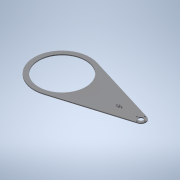
# Autodesk Inventor part: ForeArm_inside_frame
Saved by Autodesk Inventor 2020.4 (Build 244396000, 396)
## iProperties
Created: 2016-05-04
Part Number: ForeArm_inside_frame
Material: GFRP
Document SubType Name: Modeling
Designer: hiroaki
Density: 1.75 g/cm^3
Appearance: 滑らか - 淡い灰色
Mass: 3.24569 g
Surface Area: 24.0552 cm^2
Volume: 1.85468 cm^3
Description: GFRP T2
d0: 147.500 mm
d1: 3.100 mm
d2: 21.000 mm
d3: 10.000 mm
d4: 5.000 mm
d5: 12.000 mm
d6: 100.000 mm
d7: 5.000 mm
d8: 0.050 mm
d9: 2.100 mm
d10: 2.700 mm
d11: 8.500 mm
d12: 10.100 mm
d13: 4.000 ul
d15: 360.00 deg
d17: 2.000 mm
d18: 0.00 deg
Author: hiroaki
Autodesk Inventor part; units mm, degrees
ref_plane "YZ Plane" through (0, 0, 0) normal (1, 0, 0) x (0, 1, 0)
ref_plane "XZ Plane" through (0, 0, 0) normal (0, 1, 0) x (-1, 0, 0)
ref_plane "XY Plane" through (0, 0, 0) normal (0, 0, 1) x (1, 0, 0)
sketch "スケッチ1" plane through (0, 0, 0) normal (0, 0, 1) x (1, 0, 0)
  circle A0 centre (0, 0) radius 10.5 construction
  line L0 (0, 10.5) -> (-147.5, 10.5) construction
  line L1 (-147.5, 10.5) -> (-147.5, -10.5) construction
  line L2 (-147.5, -10.5) -> (0, -10.5) construction
  circle A1 centre (-142.5, 0) radius 1.55 construction
  line L3 (-132.5, 2.5) -> (-52.5, 2.5) construction
  line L4 (-52.5, 2.5) -> (-52.5, -2.5) construction
  line L5 (-52.5, -2.5) -> (-132.5, -2.5) construction
  line L6 (-132.5, -2.5) -> (-132.5, 2.5) construction
  line L7 (-92.5, 2.5) -> (-92.5, -2.5) construction
  circle A2 centre (-42.5, 0) radius 1.55 construction
  line L8 (-12, 21.3027) -> (-12, -27.3903) construction
  line L9 (-52.45, 2.55) -> (-132.55, 2.55) construction
  line L10 (-132.55, 2.55) -> (-132.55, -2.55) construction
  line L11 (-132.55, -2.55) -> (-52.45, -2.55) construction
  line L12 (-52.45, -2.55) -> (-52.45, 2.55) construction
  circle A3 centre (-131.5, 2.55) radius 1.05 construction
  line L13 (-132.5, 0) -> (-92.5, 0) construction
  line L14 (-132.55, 2.55) -> (-132.55, -2.55) construction
  arc A4 (-130.45, 2.55) -> (-132.55, 2.55) centre (-131.5, 2.55) ccw construction
  line L15 (-130.45, 2.55) -> (-54.55, 2.55) construction
  arc A5 (-52.45, 2.55) -> (-54.55, 2.55) centre (-53.5, 2.55) ccw construction
  line L16 (-52.45, 2.55) -> (-52.45, -2.55) construction
  arc A6 (-132.55, -2.55) -> (-130.45, -2.55) centre (-131.5, -2.55) ccw construction
  line L17 (-130.45, -2.55) -> (-54.55, -2.55) construction
  arc A7 (-54.55, -2.55) -> (-52.45, -2.55) centre (-53.5, -2.55) ccw construction
  circle A8 centre (0, 8.5) radius 1.35
  circle A9 centre (0, 0) radius 5.05
  circle A10 centre (-8.5, 0) radius 1.35
  circle A11 centre (0, -8.5) radius 1.35
  circle A12 centre (8.5, 0) radius 1.35
  line L18 (-147.5, 4.7329) -> (-147.5, -4.7329) construction
  line L19 (-147.5, 4.7329) -> (-42.5, 10.5) construction
  line L20 (-42.5, 10.5) -> (0, 10.5) construction
  line L21 (-147.5, -4.7329) -> (-42.5, -10.5) construction
  line L22 (-42.5, -10.5) -> (0, -10.5) construction
  arc A13 (0, -10.5) -> (0, 10.5) centre (0, 0) ccw construction
  circle A14 centre (-142.5, 0) radius 5 construction
  circle A15 centre (-41.5, 0) radius 1.55
  circle A16 centre (-51.5, 0) radius 1.55
  line L23 (-37.5, -2.5) -> (-55.5, -2.5) construction
  line L24 (-55.5, -2.5) -> (-55.5, 2.5) construction
  line L25 (-55.5, 2.5) -> (-37.5, 2.5) construction
  line L26 (-37.5, 2.5) -> (-37.5, -2.5) construction
  line L27 (-47.5, -2.5) -> (-45.5, -2.5) construction
  line L28 (-45.5, -2.5) -> (-45.5, 2.5) construction
  line L29 (-45.5, 2.5) -> (-47.5, 2.5) construction
  line L30 (-47.5, 2.5) -> (-47.5, -2.5) construction
  line L31 (-47.45, -2.55) -> (-45.55, -2.55)
  line L32 (-45.55, -2.55) -> (-45.55, 2.55)
  line L33 (-45.55, 2.55) -> (-47.45, 2.55)
  line L34 (-47.45, 2.55) -> (-47.45, -2.55)
  circle A17 centre (-48.5, -2.55) radius 1.05
  circle A18 centre (-48.5, 2.55) radius 1.05
  circle A19 centre (-44.5, -2.55) radius 1.05
  circle A20 centre (-44.5, 2.55) radius 1.05
  line L35 (-55.5, 2.5) -> (-55.5, -2.5)
  line L36 (-55.5, -2.5) -> (-21.9113, -10.5)
  line L37 (-55.5, 2.5) -> (-21.9113, 10.5)
  arc A21 (0, -10.5) -> (0, 10.5) centre (0, 0) ccw
  line L38 (-21.9113, 10.5) -> (0, 10.5)
  line L39 (0, -10.5) -> (-21.9113, -10.5)
  circle A22 centre (-44.5, 2.55) radius 2.5 construction
  circle A23 centre (0, 0) radius 16 construction
  circle A24 centre (0, 0) radius 21 construction
  line L40 (-21, 19.3585) -> (-21, -28.09) construction
  circle A25 centre (-169.122, 0) radius 50.4075
  circle A26 centre (-169.122, 0) radius 60
  line L41 (-151.5607, 57.3725) -> (3.0732, 10.0402)
  line L42 (-151.5607, -57.3725) -> (3.0732, -10.0402)
  point P0 (-147.5, 0)
  point P1 (-37.5, 0)
  point P2 (3.0732, -10.0402)
  dimension "d9" = 2.1
  dimension "d29" = 2.1
  dimension "d36" = 120
  dimension "d0" = 147.5
  dimension "d1" = 3.1
  dimension "d2" = 21
  dimension "d3" = 10
  dimension "d4" = 5
  dimension "d5" = 12
  dimension "d6" = 100
  dimension "d7" = 5
  dimension "d8" = 0.05
  dimension "d10" = 2.7
  dimension "d11" = 8.5
  dimension "d12" = 10.1
  dimension "d15" = 360
  dimension "d20" = 3.1
  dimension "d21" = 5
  dimension "d22" = 4
  dimension "d23" = 5
  dimension "d24" = -10
  dimension "d26" = 10
  dimension "d27" = 4
  dimension "d28" = 10
  dimension "d30" = 0.05
  dimension "d32" = 5
  dimension "d33" = 32
  dimension "d34" = 5
  dimension "d35" = 100.815
  dimension "d37" = 169.122
  constraints: 86 end point, 20 centre point, 15 point on circle, 12 tangent, 11 horizontal alignment, 10 coincident, 10 parallel, 9 horizontal, 8 perpendicular, 7 midpoint, 7 symmetric about line, 6 point on line, 5 collinear, 5 vertical, 4 equal radius, 3 vertical alignment, 2 concentric, 34 other
  measures "d0" distance from line of L1 point (0, 0)
  measures "d1" diameter of A1
  measures "d2" distance of L0.end L1.end
  measures "d3" distance from line of L6 A1.centre
  measures "d4" distance from line of L1 A1.centre
  measures "d5" distance from line of point (0, 0) L8
  measures "d6" distance of A2.centre A1.centre
  measures "d7" distance of L3.end L4.end
  measures "d8" distance between parallel lines of L9 L3
  measures "d10" diameter of A8
  measures "d11" distance of point (0, 0) A8.centre
  measures "d12" diameter of A9
  measures "d20" diameter of A15
  measures "d21" distance from line of L26 A2.centre
  measures "d22" distance from line of L26 A15.centre
  measures "d23" distance of L25.end L23.start
  measures "d24" distance of A16.centre A15.centre
  measures "d26" distance between parallel lines of L30 L26
  measures "d27" distance from line of A16.centre L24
  measures "d28" distance between parallel lines of L28 L24
  measures "d30" distance between parallel lines of L34 L30
  measures "d32" diameter of A22
  measures "d33" diameter of A23
  measures "d34" radial gap between concentric circles of A24 A23
  measures "d35" diameter of A25
  measures "d37" distance of point (0, 0) A25.centre
extrude "押し出し1" add sketch "スケッチ1" along normal blind 2
fillet "フィレット2" [suppressed]
equation "\"d0\" = d0_1"
equation "\"d2\" = d2_1"
equation "\"d3\" = d3_1"
equation "\"d4\" = d4_1"
equation "\"d6\" = d6_1"
equation "\"d21\" = d4"
equation "\"d27\" = d22"
equation "\"d28\" = d26"
equation "\"d2_1\" = 21"
equation "\"d3_1\" = 10"
equation "\"d4_1\" = 5"
equation "\"d6_1\" = 100"
equation "\"d0_1\" = 147.5"
